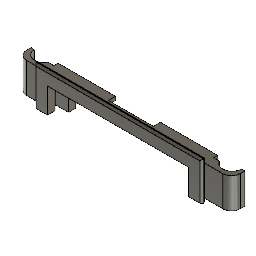
panelling top (Autodesk Fusion 360 design; units mm, degrees)
Autodesk Fusion 360 part; units mm, degrees
sketch "Skizze1" plane through (0, 0, 0) normal (0, 0, 1) x (1, 0, 0)
  line L0 (0, 0) -> (39.9, 0) construction
  circle A0 centre (39.9, 0) radius 3.8
  line L1 (33.05, -7.2) -> (46.9, -7.2)
  line L2 (46.9, -7.2) -> (46.9, 42.9968)
  line L3 (45.6, -5.9) -> (45.6, 33.959)
  line L4 (45.6, -5.9) -> (33.05, -5.9)
  line L5 (36.733, 2.1) -> (30.2653, 2.1)
  line L6 (30.2653, 2.1) -> (30.2653, -2.1)
  line L7 (30.2653, -2.1) -> (36.733, -2.1)
  line L8 (36.733, -2.1) -> (36.733, 2.1)
  arc A1 (41.6, -5.9) -> (45.6, -1.9) centre (41.6, -1.9) ccw
  line L9 (43.9, 0) -> (45.4, 0)
  line L10 (45.4, 0) -> (45.4, -1.9)
  arc A2 (36.6274, -2.3) -> (43.9, 0) centre (39.9, 0) ccw
  arc A3 (41.6, -5.7) -> (45.4, -1.9) centre (41.6, -1.9) ccw
  line L11 (41.6, -5.7) -> (32.85, -5.7)
  line L12 (36.6274, -2.3) -> (0, -2.3)
  line L13 (33.05, -7.2) -> (33.05, -5.9)
  line L14 (32.85, -5.7) -> (32.85, -7.3)
  line L15 (32.85, -7.3) -> (35.55, -7.3)
  line L16 (35.55, -7.3) -> (35.55, -8.5)
  line L17 (35.55, -8.5) -> (0, -8.5)
  line L18 (0, -2.3) -> (0, -8.5)
  dimension "d1" = 39.9
  dimension "d2" = 7.6
  dimension "d3" = 7.2
  dimension "d5" = 1.3
  dimension "d6" = 1.3
  dimension "d7" = 4.2
  dimension "d8" = 4
  dimension "d10" = 0.2
  dimension "d11" = 0.2
  dimension "d12" = 0.2
  dimension "d13" = 0.2
  dimension "d14" = 0.2
  dimension "d15" = 33.05
  dimension "d16" = 0.2
  dimension "d17" = 0.1
  dimension "d18" = 2.7
  dimension "d19" = 1.2
  dimension "d47" = 7
  constraint coincident L0.start origin
  constraint horizontal L0
  constraint coincident L0.end A0.centre
  constraint horizontal L1
  constraint perpendicular L1 L2
  constraint vertical L3
  constraint perpendicular L3 L4
  constraint horizontal L5
  constraint vertical L6
  constraint horizontal L7
  constraint vertical L8
  constraint coincident A0 L5.start
  constraint coincident A0 L7.end
  constraint tangent L3 A1
  constraint coincident L3 A1.end
  constraint coincident L4 A1.start
  constraint tangent L4 A1
  constraint horizontal L9
  constraint perpendicular L9 L10
  constraint horizontal L11
  constraint horizontal L12
  constraint concentric A0 A2
  constraint concentric A1 A3
  constraint collinear L0 L9
  constraint perpendicular L4 L13
  constraint perpendicular L11 L14
  constraint perpendicular L14 L15
  constraint perpendicular L15 L16
  constraint perpendicular L16 L17
  constraint perpendicular L17 L18
  measures "d1" distance of L0.start L0.end
  measures "d2" diameter of A0
  measures "d3" distance of L0.end L1
  measures "d5" distance of L2 L3
  measures "d6" distance of L1 L4
  measures "d7" distance of L5.start L7.end
  measures "d8" distance of L3.start A1.end
  measures "d10" distance of A1 A3
  measures "d11" distance of L3 L10
  measures "d12" distance of A0 A2
  measures "d13" distance of L7 L12
  measures "d14" distance of L4 L11
  measures "d15" distance of L0.start L13
  measures "d16" distance of L13 L14
  measures "d17" distance of L1 L15
  measures "d18" distance of L14.end L15.end
  measures "d19" distance of L15.end L16.end
  measures "d47" distance of L2 L0.end
extrude "Extrusion1" add sketch "Skizze1" along normal blind 16.4 contours L9 L10 A2 A3 L11 L12 L14 L15 L16 L17 L18
sketch "Skizze2" plane through (0, 0, 0) normal (0, 0, -1) x (1, 0, 0)
  line L0 (0, 2.3) -> (36.6274, 2.3)
  arc A0 (43.9, 0) -> (36.6274, 2.3) centre (39.9, 0) ccw
  line L1 (43.9, 0) -> (45.4, 0)
  line L2 (45.4, 0) -> (45.4, 1.9)
  arc A1 (45.4, 1.9) -> (41.6, 5.7) centre (41.6, 1.9) ccw
  line L3 (41.6, 5.7) -> (32.85, 5.7)
  line L4 (32.85, 5.7) -> (32.85, 7.3)
  line L5 (32.85, 7.3) -> (35.55, 7.3)
  line L6 (35.55, 7.3) -> (35.55, 8.5)
  line L7 (35.55, 8.5) -> (0, 8.5)
  line L8 (0, 8.5) -> (0, 2.3)
  line L9 (32.85, 5.2) -> (32.85, 3)
  line L10 (32.85, 5.2) -> (29.95, 5.2)
  line L11 (29.95, 5.2) -> (29.95, 8.5)
  line L12 (32.85, 3) -> (26.45, 3)
  line L13 (26.45, 3) -> (26.45, 2.3)
  line L14 (32.85, 3) -> (32.85, 2.3) construction
  arc A2 (34.05, 2.3) -> (32.85, 5.2) centre (17.5457, -2.8311) ccw
  dimension "d23" = 3.3
  dimension "d24" = 2.2
  dimension "d25" = 32.85
  dimension "d26" = 2.9
  dimension "d27" = 6.4
  dimension "d34" = 1.2
  constraint perpendicular L9 L10
  constraint coincident L7 L11.end
  constraint perpendicular L7 L11
  constraint perpendicular L9 L12
  constraint coincident L0 L13.end
  constraint perpendicular L0 L13
  constraint coincident L0 L14.end
  constraint perpendicular L0 L14
  constraint coincident L0 A2.start
  measures "d23" distance of L7 L10
  measures "d24" distance of L9.start L9.end
  measures "d25" distance of L8 L9
  measures "d26" distance of L9.start L10.end
  measures "d27" distance of L9.end L12.end
  measures "d34" distance of L14.end A2.start
extrude "Extrusion2" cut sketch "Skizze2" against normal blind 10.8 contours L0 L7 L8 L9 L10 L11 L12 L13
sketch "Skizze3" plane through (0, 0, 10.8) normal (0, 0, -1) x (1, 0, 0)
  line L0 (32.85, 5.2) -> (29.95, 5.2)
  line L1 (29.95, 5.2) -> (29.95, 8.5)
  line L2 (29.95, 8.5) -> (0, 8.5)
  line L3 (0, 8.5) -> (0, 2.3)
  line L4 (0, 2.3) -> (26.45, 2.3)
  line L5 (26.45, 2.3) -> (26.45, 3)
  line L6 (26.45, 3) -> (32.85, 3)
  line L7 (32.85, 3) -> (32.85, 5.2)
  line L8 (29.95, 5.2) -> (0, 5.2)
  line L9 (26.45, 3) -> (0, 3)
  constraint coincident L0.end L1.start
  constraint coincident L3 L8.end
  constraint perpendicular L3 L8
  constraint coincident L5.end L6.start
  constraint coincident L3 L9.end
  constraint perpendicular L3 L9
extrude "Extrusion3" cut sketch "Skizze3" against normal blind 0.6 contours L0 L3 L6 L7 L8 L9
mirror "Spiegeln1" about plane through (0, 0, 0) normal (1, 0, 0) of bodies 1 merged
extrude "Extrusion4" cut sketch "Skizze2" against normal blind 4.5 contours L0 L9 L12 L13 A2
sketch "Skizze5" plane through (0, 0, 10.8) normal (0, 0, -1) x (1, 0, 0)
  line L0 (26.45, 3) -> (-26.45, 3)
  line L1 (-26.45, 3) -> (-26.45, 2.3)
  line L2 (-26.45, 2.3) -> (26.45, 2.3)
  line L3 (26.45, 2.3) -> (26.45, 3)
  line L4 (-9.5, 2.3) -> (9.5, 2.3)
  line L5 (9.5, 2.3) -> (9.5, 3)
  line L6 (9.5, 3) -> (-9.5, 3)
  line L7 (-9.5, 3) -> (-9.5, 2.3)
  dimension "d39" = 19
  constraint horizontal L4
  constraint vertical L5
  constraint horizontal L6
  constraint vertical L7
  constraint coincident L0 L5.end
  constraint coincident L2 L4.start
  constraint midpoint L2 L4
  measures "d39" distance of L5.end L6.end
extrude "Extrusion6" cut sketch "Skizze5" against normal blind 4.6 contours L0 L2 L4 L5 L6 L7
sketch "Skizze6" plane through (0, 0, 16.4) normal (0, 0, 1) x (-1, 0, 0)
  line L0 (-36.6274, 2.3) -> (36.6274, 2.3)
  arc A0 (43.9, 0) -> (36.6274, 2.3) centre (39.9, 0) ccw
  line L1 (43.9, 0) -> (45.4, 0)
  line L2 (45.4, 0) -> (45.4, 1.9)
  arc A1 (45.4, 1.9) -> (41.6, 5.7) centre (41.6, 1.9) ccw
  line L3 (41.6, 5.7) -> (32.85, 5.7)
  line L4 (32.85, 5.7) -> (32.85, 7.3)
  line L5 (32.85, 7.3) -> (35.55, 7.3)
  line L6 (35.55, 7.3) -> (35.55, 8.5)
  line L7 (35.55, 8.5) -> (-35.55, 8.5)
  line L8 (-35.55, 8.5) -> (-35.55, 7.3)
  line L9 (-35.55, 7.3) -> (-32.85, 7.3)
  line L10 (-32.85, 7.3) -> (-32.85, 5.7)
  line L11 (-32.85, 5.7) -> (-41.6, 5.7)
  arc A2 (-41.6, 5.7) -> (-45.4, 1.9) centre (-41.6, 1.9) ccw
  line L12 (-45.4, 1.9) -> (-45.4, 0)
  line L13 (-45.4, 0) -> (-43.9, 0)
  arc A3 (-36.6274, 2.3) -> (-43.9, 0) centre (-39.9, 0) ccw
  line L14 (32.85, 7.3) -> (-32.85, 7.3)
  line L15 (32.85, 5.7) -> (-32.85, 5.7)
  constraint coincident L4.end L5.start
  constraint coincident L9.end L10.start
  constraint coincident L3.end L4.start
  constraint coincident L10.end L11.start
extrude "Extrusion7" cut sketch "Skizze6" against normal blind 3.4 contours L4 L10 L14 L15
extrude "Extrusion8" cut 1 faces at (-12.6469, -4.9624, 16.4) along direction (0, 0, -1) blind 3.4
chamfer "Fase1" distance 0.8 angle 45 3 edges at (35.55, -8.5, 8.2) (0, -8.5, 16.4) (-35.55, -8.5, 8.2)
chamfer "Fase1" distance 0.6 angle 45 2 edges at (9.5, -2.65, 10.8) (-9.5, -2.65, 10.8)
fillet "Abrundung1" radius 2.4 2 edges at (-32.85, -4.1, 11.4) (32.85, -4.1, 11.4)
move_face "Flächen versetzen1" offset 0.5 2 faces at (32.3758, -2.3, 9.4333) (-33.2349, -2.3, 7.9333)
sketch "Skizze7" plane through (0, -1.8, 0) normal (0, 1, 0) x (-1, 0, 0)
  line L0 (9.5, 11.4) -> (10.1, 10.8)
  line L1 (10.1, 10.8) -> (26.45, 10.8)
  line L2 (26.45, 10.8) -> (26.45, 0)
  line L3 (26.45, 0) -> (36.3279, 0)
  line L4 (36.3279, 0) -> (36.3279, 13)
  line L5 (36.3279, 13) -> (9.5, 13)
  line L6 (9.5, 13) -> (9.5, 11.4)
  line L7 (33.9, 13) -> (33.9, 0)
  line L8 (-10.1, 10.8) -> (-9.5, 11.4)
  line L9 (-9.5, 11.4) -> (-9.5, 13)
  line L10 (-9.5, 13) -> (-36.3279, 13)
  line L11 (-36.3279, 13) -> (-36.3279, 0)
  line L12 (-36.3279, 0) -> (-34.1972, 0)
  line L13 (-34.1972, 0) -> (-34.1972, 4.5)
  line L14 (-34.1972, 4.5) -> (-26.45, 4.5)
  line L15 (-26.45, 4.5) -> (-26.45, 10.8)
  line L16 (-26.45, 10.8) -> (-10.1, 10.8)
  line L17 (-33.9, 13) -> (-33.9, 4.5)
  point P0 (43.9, 13)
  point P1 (-43.9, 13)
  dimension "d52" = 10
  dimension "d53" = 10
  constraint coincident L5 L7.start
  constraint coincident L3 L7.end
  constraint perpendicular L3 L7
  constraint coincident L10 L17.start
  constraint perpendicular L10 L17
  constraint coincident L14 L17.end
  measures "d52" distance of L7.start P0
  measures "d53" distance of L17.start P1
extrude "Extrusion9" add sketch "Skizze7" along normal blind 1.8 contours L0 L1 L2 L3 L5 L6 L7 | L8 L9 L10 L14 L15 L16 L17
equation "d1 = ( 79.8 / 2 ) * 1 mm"
equation "d3 = 11 mm - ( 7.6 / 2 ) * 1 mm"
equation "toleranz = 0.2 mm"
equation "d10 = toleranz"
equation "d11 = toleranz"
equation "d12 = toleranz"
equation "d13 = toleranz"
equation "d14 = toleranz"
equation "d15 = ( 66.1 / 2 ) * 1 mm"
equation "d16 = toleranz"
equation "d25 = ( 65.7 / 2 ) * 1 mm"
equation "d28 = -10.7 mm + 0.6 mm - 0.7 mm"
equation "d40 = -4.00 mm - 0.6 mm"
